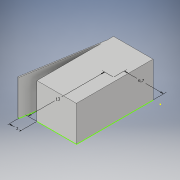
# Autodesk Inventor part: koncnostikalo
Saved by Autodesk Inventor 2019 (Build 230136000, 136)
## iProperties
Created: 2020-07-29
Part Number: koncnostikalo
Material: Generic
Document SubType Name: Modeling
Designer: lukad
Density: 1 g/cm^3
Appearance: Default
Author: lukad
Autodesk Inventor part; units mm, degrees
ref_plane "YZ Plane" through (0, 0, 0) normal (1, 0, 0) x (0, 1, 0)
ref_plane "XZ Plane" through (0, 0, 0) normal (0, 1, 0) x (-1, 0, 0)
ref_plane "XY Plane" through (0, 0, 0) normal (0, 0, 1) x (1, 0, 0)
sketch "Sketch1" plane through (0, 0, 0) normal (0, 1, 0) x (-1, 0, 0)
  line L0 (1.2588, 13) -> (7.9588, 13)
  line L1 (7.9588, 13) -> (7.9588, 0)
  line L2 (7.9588, 0) -> (1.2588, 0)
  line L3 (1.2588, 0) -> (1.2588, 13)
  line L4 (7.9588, 1.0722) -> (10.1386, 14.0497)
  line L5 (10.1386, 14.0497) -> (9.9588, 14.0799)
  line L6 (9.9588, 14.0799) -> (7.9588, 2.173)
  point P0 (0, 0)
  dimension "d0" = 13
  dimension "d1" = 6.7
  dimension "d2" = 2
  constraints: 14 end point, 3 perpendicular, 2 parallel, 2 point on line, 1 horizontal
  measures "d0" distance of L0.end L1.end
  measures "d1" distance of L1.end L2.end
  measures "d2" horizontal distance of L0.end L5.end
extrude "Extrusion1" add sketch "Sketch1" along normal blind 6 contours L0 L1 L2 L3
extrude "Extrusion2" add sketch "Sketch1" along normal blind 6 contours L6 L5 L4 L1
body "Solid1"
